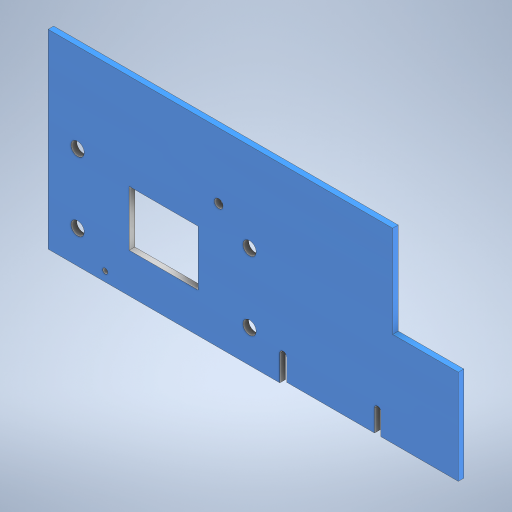
# Autodesk Inventor part: daughterboard
Saved by Autodesk Inventor 2024 (Build 280153000, 153)
## iProperties
Created: 2024-09-23
Part Number: daughterboard
Material: Generic
Document SubType Name: Modeling
Designer: PC
Density: 1 g/cm^3
Appearance: Default
Author: PC
Autodesk Inventor part; units mm, degrees
ref_plane "YZ Plane" through (0, 0, 0) normal (1, 0, 0) x (0, 1, 0)
ref_plane "XZ Plane" through (0, 0, 0) normal (0, 1, 0) x (-1, 0, 0)
ref_plane "XY Plane" through (0, 0, 0) normal (0, 0, 1) x (1, 0, 0)
sketch "Sketch1" plane through (0, 0, 0) normal (0, 0, 1) x (1, 0, 0)
  line L0 (0, 0) -> (125, 0)
  line L1 (125, 1.2) -> (125, 30)
  line L2 (105, 58) -> (0, 58)
  line L3 (0, 58) -> (0, 0)
  line L4 (105, 58) -> (105, 30)
  line L5 (105, 30) -> (125, 30)
  line L6 (24.7, 28.9) -> (45.7, 28.9)
  line L7 (45.7, 28.9) -> (45.7, 12.05)
  line L8 (45.7, 12.05) -> (24.7, 12.05)
  line L9 (24.7, 12.05) -> (24.7, 28.9)
  circle A0 centre (9, 10) radius 2
  circle A1 centre (61.4, 10) radius 2
  circle A2 centre (9, 30.95) radius 2
  circle A3 centre (61.4, 30.95) radius 2
  line L10 (9, 30.95) -> (9, 10) construction
  line L11 (9, 10) -> (61.4, 10) construction
  line L12 (70.6, 0) -> (70.6, 1.2)
  arc A4 (72.7, 7.8) -> (70.6, 7.8) centre (71.65, 7.8) ccw
  line L13 (70.6, 7.8) -> (70.6, 1.2)
  line L14 (72.7, 7.8) -> (72.7, 1.2)
  arc A5 (101.4226, 7.8) -> (99.4774, 7.8) centre (100.45, 7.8) ccw
  line L15 (99.4774, 7.8) -> (99.4774, 1.2)
  line L16 (101.4226, 7.8) -> (101.4226, 1.2)
  line L17 (72.7, 1.2) -> (99.4774, 1.2)
  line L18 (101.4226, 1.2) -> (125, 1.2)
  circle A6 centre (52, 38) radius 1.3
  circle A7 centre (17.4, 2.9) radius 0.75
  point P0 (35.2, 12.05)
  point P1 (35.2, 10)
  point P2 (9, 20.475)
  point P3 (24.7, 20.475)
  dimension "d2" = 20
  dimension "d3" = 28
  dimension "d4" = 125
  dimension "d5" = 21
  dimension "d9" = 52.4
  dimension "d12" = 20.95
  dimension "d15" = 10
  dimension "d16" = 9
  dimension "d17" = 4
  dimension "d18" = 1.2
  dimension "d19" = 54.4
  dimension "d20" = 7.8
  dimension "d21" = 2.1
  dimension "d24" = 28.8
  dimension "d27" = 2.6
  dimension "d28" = 1.5
  dimension "d29" = 2.9
  dimension "d31" = 16.85
  dimension "d33" = 34.6
  dimension "d34" = 8.4
  dimension "d35" = 35.1
  dimension "d36" = 28.8
  dimension "d37" = 26.7773
  constraints: 38 end point, 11 perpendicular, 8 centre point, 5 coincident, 4 horizontal, 4 midpoint, 4 parallel, 4 point on circle, 3 tangent, 3 vertical, 1 horizontal alignment, 1 point on line, 1 vertical alignment, 6 other
  measures "d2" distance of L1.end L4.end
  measures "d3" distance of L2.start L4.end
  measures "d4" distance between parallel lines of L3 L1
  measures "d5" distance of L6.start L6.end
  measures "d9" distance of L10.end L11.end
  measures "d12" distance of L10.end L10.start
  measures "d15" distance from line of L0 L10.end
  measures "d16" distance from line of L3 L10.start
  measures "d17" diameter of A2
  measures "d18" distance of L12.start L12.end
  measures "d19" distance of L1.start L12.end
  measures "d20" vertical distance of L12.start A4.centre
  measures "d21" diameter of A4
  measures "d24" distance of A4.centre A5.centre
  measures "d27" diameter of A6
  measures "d28" diameter of A7
  measures "d29" distance from line of L0 A7.centre
  measures "d31" distance of L6.start L8.end
  measures "d33" horizontal distance of A7.centre A6.centre
  measures "d34" horizontal distance of A7.centre L10.end
  measures "d35" vertical distance of A7.centre A6.centre
  measures "d36" distance of L1.end L1.start
  measures "d37" distance of L14.end L15.end
extrude "Extrusion1" add sketch "Sketch1" along normal blind 1.7
body "Solid1"
